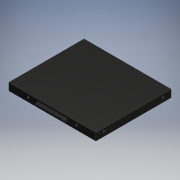
# Autodesk Inventor part: Structure_-Z
Saved by Autodesk Inventor 2018 (Build 220112000, 112)
## iProperties
Created: 2018-07-04
Part Number: Structure_-Z
Material: Aluminum 6061
Document SubType Name: Modeling
Designer: Bradley
Density: 2.7 g/cm^3
Appearance: Anodized - Dark Gray
Mass: 130.923 g
Surface Area: 191.623 cm^2
Volume: 48.49 cm^3
Author: Bradley
Autodesk Inventor part; units mm, degrees
ref_plane "YZ Plane" through (0, 0, 0) normal (1, 0, 0) x (0, 1, 0)
ref_plane "XZ Plane" through (0, 0, 0) normal (0, 1, 0) x (-1, 0, 0)
ref_plane "XY Plane" through (0, 0, 0) normal (0, 0, 1) x (1, 0, 0)
sketch "Sketch1" plane through (0, 0, 0) normal (0, 0, 1) x (1, 0, 0)
  line L0 (48, -41.5) -> (-48, -41.5)
  line L1 (-48, -41.5) -> (-48, 41.5)
  line L2 (-48, 41.5) -> (48, 41.5)
  line L3 (48, 41.5) -> (48, -41.5)
  line L4 (48, -41.5) -> (-48, 41.5) construction
  line L5 (-48, -41.5) -> (48, 41.5) construction
  point P0 (0, 0)
  dimension "d0" = 96
  dimension "d1" = 83
  constraints: 12 end point, 2 midpoint, 2 parallel, 1 horizontal, 1 perpendicular
  measures "d0" distance of L1.end L2.end
  measures "d1" distance of L0.end L1.end
extrude "Extrusion1" add sketch "Sketch1" along normal mid plane 8
sketch "Sketch2" plane through (-48, -41.5, 4) normal (0, -1, 0) x (1, 0, 0)
  line L0 (96, -8) -> (96, 0) projected
  line L1 (0, 0) -> (96, 0) projected
  line L2 (0, 0) -> (0, -8) projected
  line L3 (96, -8) -> (0, -8) projected
  line L4 (33, -4) -> (63, -4) construction
  line L5 (33, -5.5) -> (63, -5.5)
  line L6 (63, -2.5) -> (33, -2.5)
  arc A0 (33, -2.5) -> (33, -5.5) centre (33, -4) ccw
  arc A1 (63, -5.5) -> (63, -2.5) centre (63, -4) ccw
  point P0 (48, -4)
  dimension "d5" = 3
  dimension "d8" = 30
  constraints: 8 end point, 4 point on circle, 4 tangent, 2 centre point, 1 horizontal, 1 midpoint, 1 parallel
  measures "d5" diameter of A1
  measures "d8" distance of L4.start L4.end
extrude "Extrusion2" add sketch "Sketch2" along normal blind 3 contours A0 L6 A1 L5
sketch "Sketch3" plane through (-48, -41.5, 4) normal (0, -1, 0) x (1, 0, 0)
  arc A0 (33, -2.5) -> (33, -5.5) centre (33, -4) ccw projected
  line L0 (33, -2.5) -> (63, -2.5) projected
  arc A1 (63, -5.5) -> (63, -2.5) centre (63, -4) ccw projected
  line L1 (63, -5.5) -> (33, -5.5) projected
  line L2 (96, -8) -> (96, 0) projected
  line L3 (0, 0) -> (96, 0) projected
  line L4 (0, 0) -> (0, -8) projected
  line L5 (96, -8) -> (0, -8) projected
  line L6 (21.5, -3.5) -> (74.5, -3.5) construction
  point P0 (48, -3.5)
  point P1 (48, -8)
  dimension "d9" = 53
  dimension "d39" = 4.5
  constraints: 2 coincident, 2 end point, 2 midpoint, 1 horizontal, 1 vertical alignment
  measures "d9" distance of L6.start L6.end
  measures "d39" distance between parallel lines of L5 L6
hole "Hole1" at (-26.5, -41.5, 0.5) at (26.5, -41.5, 0.5) direction (0, 1, 0) diameter 2.459 depth 8.8 tip angle 118 thread size "M3x0.5" class "6H" standard "ANSI Metric M Profile"
mirror "Mirror1" about plane through (0, 0, 0) normal (0, 1, 0) of "Extrusion2", "Hole1"
fillet "Fillet1" radius 0.381 8 edges at (16.5, -41.5, 0) (0, -41.5, -1.5) (-16.5, -41.5, 0) (0, -41.5, 1.5) (-16.5, 41.5, 0) (0, 41.5, -1.5) (16.5, 41.5, 0) (0, 41.5, 1.5)
chamfer "Chamfer1" distance 0.5 angle 45 8 edges at (0, -44.5, 1.5) (-16.5, -44.5, 0) (0, -44.5, -1.5) (16.5, -44.5, 0) (0, 44.5, 1.5) (-16.5, 44.5, 0) (0, 44.5, -1.5) (16.5, 44.5, 0)
sketch "Sketch4" plane through (48, -41.5, 4) normal (1, 0, 0) x (0, 0, -1)
  line L0 (3, 9) -> (3, 74) construction
  line L1 (8, 83) -> (8, 0) projected
  line L2 (0, 83) -> (8, 83) projected
  line L3 (0, 0) -> (0, 83) projected
  line L4 (8, 0) -> (0, 0) projected
  line L5 (8, 83) -> (8, 0) projected
  line L6 (0, 0) -> (0, 83) projected
  point P0 (3, 41.5)
  point P1 (4, 41.5)
  dimension "d21" = 65
  dimension "d29" = 5
  constraints: 2 coincident, 2 end point, 1 horizontal alignment, 1 midpoint, 1 vertical
  measures "d21" distance of L0.start L0.end
  measures "d29" distance between parallel lines of L1 L0
hole "Hole2" at (48, -32.5, 1) at (48, 32.5, 1) direction (-1, 0, 0) diameter 2.459 depth 8.8 tip angle 118 thread size "M3x0.5" class "6H" standard "ANSI Metric M Profile"
mirror "Mirror2" about plane through (0, 0, 0) normal (1, 0, 0) of "Hole2"
body "Solid1"
